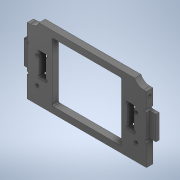
# Autodesk Inventor part: Cockpit_horizontal_frame_04
Saved by Autodesk Inventor 2020.4 (Build 244396000, 396)
## iProperties
Created: 2021-08-14
Part Number: Cockpit_horizontal_frame_04
Material: アセタール樹脂、黒
Document SubType Name: Modeling
Designer: Masato Kubotera
Density: 1.425 g/cm^3
Appearance: 滑らか - 黒
Mass: 21.2225 g
Surface Area: 93.399 cm^2
Volume: 14.8929 cm^3
Author: Masato Kubotera
Title: Cockpit_horizontal_frame_04
Autodesk Inventor part; units mm, degrees
ref_plane "YZ Plane" through (0, 0, 0) normal (1, 0, 0) x (0, 1, 0)
ref_plane "XZ Plane" through (0, 0, 0) normal (0, 1, 0) x (-1, 0, 0)
ref_plane "XY Plane" through (0, 0, 0) normal (0, 0, 1) x (1, 0, 0)
sketch "スケッチ1" plane through (0, 0, 0) normal (0, 0, 1) x (1, 0, 0)
  line L0 (-47, 28.25) -> (-37.7144, 28.25)
  line L1 (47, 28.25) -> (47, 23.75)
  line L2 (47, -28.25) -> (-47, -28.25)
  line L3 (-47, -28.25) -> (-47, -11.5167)
  line L4 (-47, 28.25) -> (47, -28.25) construction
  line L5 (47, 28.25) -> (-47, -28.25) construction
  line L6 (0, 28.25) -> (0, -28.25) construction
  line L7 (-37.25, 9.4167) -> (-32.25, 9.4167) construction
  line L8 (-32.25, 9.4167) -> (-32.25, -9.4167) construction
  line L9 (-32.25, -9.4167) -> (-37.25, -9.4167) construction
  line L10 (-37.25, -9.4167) -> (-37.25, 9.4167) construction
  line L11 (-37.25, 9.4167) -> (-32.25, -9.4167) construction
  line L12 (-32.25, 9.4167) -> (-37.25, -9.4167) construction
  line L13 (-37.3, 9.4667) -> (-32.2, 9.4667)
  line L14 (-32.2, 9.4667) -> (-32.2, 7.3667) construction
  line L15 (-32.2, -9.4667) -> (-37.3, -9.4667)
  line L16 (-37.3, -9.4667) -> (-37.3, -7.3667) construction
  line L17 (-37.3, 9.4667) -> (-32.2, -9.4667) construction
  line L18 (-32.2, 9.4667) -> (-37.3, -9.4667) construction
  arc A0 (-37.3, 9.4667) -> (-37.3, 7.3667) centre (-37.3, 8.4167) ccw
  line L19 (-34.75, 9.4667) -> (-34.75, -9.4667) construction
  arc A1 (-32.2, 7.3667) -> (-32.2, 9.4667) centre (-32.2, 8.4167) ccw
  line L20 (-37.3, 7.3667) -> (-37.3, 9.4667) construction
  line L21 (-32.2, 7.3667) -> (-32.2, -7.3667)
  line L22 (-37.3, -7.3667) -> (-37.3, 7.3667)
  line L23 (-32.2, -7.3667) -> (-32.2, -9.4667) construction
  line L24 (37.25, 9.4167) -> (32.25, 9.4167) construction
  line L25 (32.25, 9.4167) -> (32.25, -9.4167) construction
  line L26 (32.25, -9.4167) -> (37.25, -9.4167) construction
  line L27 (37.25, -9.4167) -> (37.25, 9.4167) construction
  line L28 (37.25, 9.4167) -> (32.25, -9.4167) construction
  line L29 (32.25, 9.4167) -> (37.25, -9.4167) construction
  line L30 (37.3, 9.4667) -> (32.2, 9.4667)
  line L31 (32.2, 9.4667) -> (32.2, 7.3667) construction
  line L32 (32.2, -9.4667) -> (37.3, -9.4667)
  line L33 (37.3, -9.4667) -> (37.3, -7.3667) construction
  line L34 (37.3, 9.4667) -> (32.2, -9.4667) construction
  line L35 (32.2, 9.4667) -> (37.3, -9.4667) construction
  arc A2 (37.3, 7.3667) -> (37.3, 9.4667) centre (37.3, 8.4167) ccw
  line L36 (34.75, 9.4667) -> (34.75, -9.4667) construction
  arc A3 (32.2, 9.4667) -> (32.2, 7.3667) centre (32.2, 8.4167) ccw
  line L37 (37.3, 7.3667) -> (37.3, 9.4667) construction
  line L38 (32.2, 7.3667) -> (32.2, -7.3667)
  line L39 (37.3, -7.3667) -> (37.3, 7.3667)
  line L40 (32.2, -7.3667) -> (32.2, -9.4667) construction
  line L41 (-52, 9.4167) -> (-52, -9.4167)
  line L42 (-52, 9.4167) -> (-47, 9.4167)
  arc A4 (-47, 9.4167) -> (-47, 11.5167) centre (-47, 10.4667) ccw
  line L43 (-47, 11.5167) -> (-47, 23.75)
  line L44 (-47, -11.5167) -> (-47, 11.5167)
  line L45 (52, 9.4167) -> (52, -9.4167)
  line L46 (52, 9.4167) -> (47, 9.4167)
  arc A5 (47, 11.5167) -> (47, 9.4167) centre (47, 10.4667) ccw
  line L47 (47, 11.5167) -> (47, -11.5167)
  line L48 (47, -11.5167) -> (47, -28.25)
  line L49 (-52, 0) -> (52, 0) construction
  line L50 (-52, -9.4167) -> (-47, -9.4167)
  arc A6 (-47, -11.5167) -> (-47, -9.4167) centre (-47, -10.4667) ccw
  arc A7 (47, -9.4167) -> (47, -11.5167) centre (47, -10.4667) ccw
  line L51 (52, -9.4167) -> (47, -9.4167)
  line L52 (-37.3, 0) -> (-32.2, 0) construction
  arc A8 (-37.3, -7.3667) -> (-37.3, -9.4667) centre (-37.3, -8.4167) ccw
  arc A9 (-32.2, -9.4667) -> (-32.2, -7.3667) centre (-32.2, -8.4167) ccw
  arc A10 (32.2, -7.3667) -> (32.2, -9.4667) centre (32.2, -8.4167) ccw
  arc A11 (37.3, -9.4667) -> (37.3, -7.3667) centre (37.3, -8.4167) ccw
  arc A12 (-47, 24.0838) -> (-37.7144, 28.25) centre (-44.75, 31.5) ccw
  arc A13 (37.7144, 28.25) -> (47, 24.0838) centre (44.75, 31.5) ccw
  line L53 (-47, 24.0838) -> (-47, 28.25)
  line L54 (-37.7144, 28.25) -> (47, 28.25)
  arc A14 (-37.7144, 28.25) -> (-47, 24.0838) centre (-44.75, 31.5) ccw
  arc A15 (47, 24.0838) -> (37.7144, 28.25) centre (44.75, 31.5) ccw
  line L55 (-44.75, 23.75) -> (-47, 23.75)
  line L56 (44.75, 23.75) -> (47, 23.75)
  line L57 (-47, 23.75) -> (-47, 24.0838)
  line L58 (47, 23.75) -> (47, 11.5167)
  line L59 (-27.25, 23.25) -> (27.25, 23.25)
  line L60 (27.25, 23.25) -> (27.25, -23.25)
  line L61 (27.25, -23.25) -> (-27.25, -23.25)
  line L62 (-27.25, -23.25) -> (-27.25, 23.25)
  line L63 (-27.25, 23.25) -> (27.25, -23.25) construction
  line L64 (27.25, 23.25) -> (-27.25, -23.25) construction
  line L65 (-42, 8.25) -> (42, 8.25) construction
  line L66 (42, 8.25) -> (42, -18.25) construction
  line L67 (42, -18.25) -> (-42, -18.25) construction
  line L68 (-42, -18.25) -> (-42, 8.25) construction
  line L69 (-42, 8.25) -> (42, -18.25) construction
  line L70 (42, 8.25) -> (-42, -18.25) construction
  circle A16 centre (-39, 5.25) radius 1.25
  line L71 (-42, -5) -> (42, -5) construction
  circle A17 centre (-39, -15.25) radius 1.25
  circle A18 centre (39, 5.25) radius 1.25
  circle A19 centre (39, -15.25) radius 1.25
  point P0 (0, 0)
  point P1 (-34.75, 0)
  point P2 (34.75, 0)
  point P3 (0, 0)
  point P4 (-34.75, 0)
  point P5 (-34.75, 0)
  point P6 (0, 0)
  point P7 (0, 0)
  point P8 (47, 9.4167)
  point P9 (47, 9.4167)
  point P10 (0, -5)
  point P11 (0, -5)
  dimension "d57" = 90
  dimension "d0" = 94
  dimension "d1" = 56.5
  dimension "d2" = 5
  dimension "d3" = 18.8333
  dimension "d4" = 1.05
  dimension "d5" = 0.05
  dimension "d6" = 0.05
  dimension "d7" = 64.5
  dimension "d10" = 1.05
  dimension "d11" = 5
  dimension "d34" = 18.8333
  dimension "d40" = 31.5
  dimension "d41" = 89.5
  dimension "d42" = 15.5
  dimension "d43" = 52
  dimension "d60" = 5
  dimension "d63" = 5
  dimension "d69" = 5
  dimension "d70" = 20
  dimension "d71" = 10
  dimension "d72" = 84
  dimension "d73" = 26.5
  dimension "d78" = 2.5
  dimension "d80" = 3
  dimension "d81" = 3
  constraints: 144 end point, 39 symmetric about line, 38 parallel, 34 point on circle, 33 midpoint, 21 perpendicular, 20 centre point, 12 point on line, 6 horizontal, 1 tangent, 1 vertical, 14 other
  measures "d0" distance of L2.start L2.end
  measures "d1" distance of L2.start L1.start
  measures "d2" distance of L8.end L9.end
  measures "d3" distance of L7.end L8.end
  measures "d4" radius of A0
  measures "d5" distance from line of L7 L19.start
  measures "d6" distance between parallel lines of L10 L22
  measures "d7" distance between parallel lines of L25 L8
  measures "d10" radius of A4
  measures "d11" horizontal distance of L41.start L0.start
  measures "d34" distance of L41.start L41.end
  measures "d40" vertical distance of L49.start A12.centre
  measures "d41" distance of A13.centre A12.centre
  measures "d42" diameter of A12
  measures "d43" distance of L2.start L1.end
  measures "d60" distance from line of L6.start L59
  measures "d63" distance between parallel lines of L62 L8
  measures "d69" distance between parallel lines of L68 L44
  measures "d70" distance between parallel lines of L54 L65
  measures "d71" vertical distance of L2.end L67.end
  measures "d72" distance of L65.start L65.end
  measures "d73" distance of L67.end L65.start
  measures "d78" diameter of A16
  measures "d80" horizontal distance of L65.start A16.centre
  measures "d81" horizontal distance of L65.start A16.centre
extrude "押し出し1" add sketch "スケッチ1" along normal blind 5 contours L54 A13 L56 L58 A5 L47 A7 L48 L2 L3 A6 L44 A4 L43 L55 A12
extrude "押し出し2" add sketch "スケッチ1" along normal blind 2.5 contours L44 L50 L41 L42 | L46 L45 L51 L47
sketch "スケッチ2" plane through (47, 11.5167, 0) normal (1, 0, 0) x (0, 0, -1)
  line L0 (0, -23.0333) -> (-5, -23.0333) projected
  line L1 (-2.5, -23.0333) -> (-2.5, -39.7667)
  line L2 (0, -39.7667) -> (-5, -39.7667) projected
  line L3 (0, -2.1) -> (-2.5, -2.1) projected
  line L4 (0, -20.9333) -> (-2.5, -20.9333) projected
  point P0 (0, -11.5167)
  point P1 (-2.5, 7.9)
  dimension "d67" = 10
  constraints: 2 end point, 2 midpoint, 1 point on line
  measures "d67" distance from line of point (-2.5, 7.9) L3
hole "穴1" at (47, 19.4167, 2.5) direction (-1, 0, 0) diameter 2.459 depth 10 tip angle 118 thread size "M3x0.5" class "6H" standard "ANSI Metric M Profile"
sketch "スケッチ3" plane through (-47, 11.5167, 0) normal (-1, 0, 0) x (0, 0, 1)
  circle A0 centre (2.5, 7.9) radius 1.2295 projected
  circle A1 centre (2.5, -30.9333) radius 1.2295 projected
  point P0 (0, -11.5167)
  point P1 (2.5, 7.9)
  constraints: 1 coincident
hole "穴2" at (-47, 19.4167, 2.5) direction (1, 0, 0) diameter 2.459 depth 10 tip angle 118 thread size "M3x0.5" class "6H" standard "ANSI Metric M Profile"
fillet "フィレット1" radius 1 4 edges at (-27.25, 23.25, 2.5) (-27.25, -23.25, 2.5) (27.25, -23.25, 2.5) (27.25, 23.25, 2.5)
equation "\"d3\" = d34"
equation "\"d6\" = d5"
equation "\"d10\" = d4"
